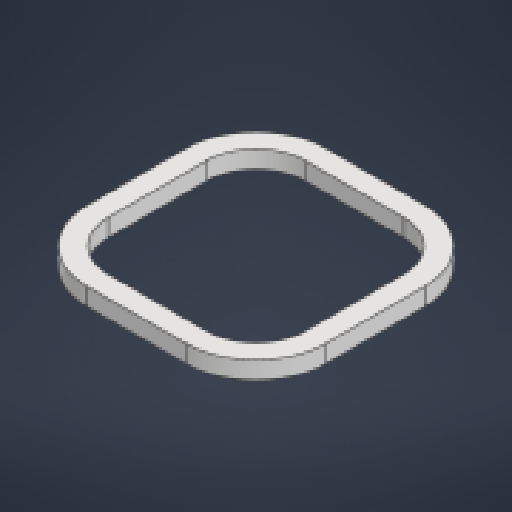
# Autodesk Inventor part: tenzo
Saved by Autodesk Inventor 2024 (Build 280153000, 153)
## iProperties
Created: 2024-06-29
Part Number: tenzo
Material: Generic
Document SubType Name: Modeling
Designer: markm
Density: 1 g/cm^3
Appearance: Default
Author: markm
Autodesk Inventor part; units mm, degrees
ref_plane "YZ Plane" through (0, 0, 0) normal (1, 0, 0) x (0, 1, 0)
ref_plane "XZ Plane" through (0, 0, 0) normal (0, 1, 0) x (-1, 0, 0)
ref_plane "XY Plane" through (0, 0, 0) normal (0, 0, 1) x (1, 0, 0)
sketch "Sketch1" plane through (0, 0, 0) normal (0, 1, 0) x (-1, 0, 0)
  line L0 (-7, 17) -> (7, 17)
  line L1 (17, 7) -> (17, -7)
  line L2 (7, -17) -> (-7, -17)
  line L3 (-17, -7) -> (-17, 7)
  line L4 (-17, 17) -> (17, -17) construction
  line L5 (17, 17) -> (-17, -17) construction
  arc A0 (7, -17) -> (17, -7) centre (7, -7) ccw
  arc A1 (-17, -7) -> (-7, -17) centre (-7, -7) ccw
  arc A2 (-7, 17) -> (-17, 7) centre (-7, 7) ccw
  arc A3 (17, 7) -> (7, 17) centre (7, 7) ccw
  line L6 (14, -7) -> (14, 7)
  arc A4 (14, 7) -> (7, 14) centre (7, 7) ccw
  line L7 (7, 14) -> (-7, 14)
  arc A5 (-7, 14) -> (-14, 7) centre (-7, 7) ccw
  line L8 (-14, 7) -> (-14, -7)
  arc A6 (-14, -7) -> (-7, -14) centre (-7, -7) ccw
  line L9 (-7, -14) -> (7, -14)
  arc A7 (7, -14) -> (14, -7) centre (7, -7) ccw
  point P0 (0, 0)
  dimension "d0" = 34
  dimension "d1" = 10
  dimension "d2" = 3
  constraints: 20 end point, 16 point on circle, 8 centre point, 8 point on line, 8 tangent, 4 parallel, 3 equal radius, 3 perpendicular, 2 midpoint, 1 horizontal, 7 other
  measures "d0" distance of L5.start L4.end
  measures "d1" radius of A0
  measures "d2" distance between parallel lines of L1 L6
extrude "Extrusion1" add sketch "Sketch1" along normal mid plane 7.75
body "Solid1"
